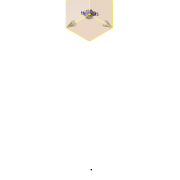
# Autodesk Inventor part: CounterWeightFixation_oldVersion
Saved by Autodesk Inventor 2021.4 (Build 254397000, 397)
## iProperties
Created: 2022-07-01
Part Number: CounterWeightFixation_oldVersion
Material: PAEK Plastic
Document SubType Name: Modeling
Designer: alexw
Density: 0.206549 g/cm^3
Appearance: Smooth - White
Mass: 22 g
Surface Area: 255.397 cm^2
Volume: 106.513 cm^3
Author: alexw
Autodesk Inventor part; units mm, degrees
ref_plane "YZ Plane" through (0, 0, 0) normal (1, 0, 0) x (0, 1, 0)
ref_plane "XZ Plane" through (0, 0, 0) normal (0, 1, 0) x (-1, 0, 0)
ref_plane "XY Plane" through (0, 0, 0) normal (0, 0, 1) x (1, 0, 0)
sketch "Sketch1" plane through (0, 0, 0) normal (0, 0, 1) x (1, 0, 0)
  arc A0 (0, 30) -> (0, -30) centre (0, 0) ccw
  arc A1 (0, 17.5) -> (0, -17.5) centre (0, 0) ccw
  line L0 (0, 36.2) -> (0, -36.2) construction
  line L1 (0, 17.5) -> (0, 36.2) construction
  line L2 (0, -17.5) -> (0, -36.2) construction
  circle A2 centre (-74.9655, 11.8734) radius 20.1
  circle A3 centre (0, 0) radius 75.9 construction
  arc A4 (0, 23.75) -> (0, -23.75) centre (0, 0) ccw construction
  line L3 (0, -23.75) -> (0, 23.75) construction
  line L4 (0, 23.75) -> (0, 0) construction
  arc A5 (0, 17.5) -> (0, 36.2) centre (0, 26.85) ccw
  arc A6 (0, -36.2) -> (0, -17.5) centre (0, -26.85) ccw
  arc A7 (-75.423, 35.4689) -> (-88.8905, -7.1807) centre (-74.9655, 11.8734) ccw
  line L5 (0, 30) -> (8.8034, 30)
  line L6 (0, -30) -> (8.8034, -30)
  arc A8 (0, 36.2) -> (0, -36.2) centre (0, 0) ccw
  circle A9 centre (-74.9655, 11.8734) radius 23.6 construction
  arc A10 (0, 36.2) -> (-75.423, 35.4689) centre (0, -3854.8474) ccw
  arc A11 (-88.8905, -7.1807) -> (0, -36.2) centre (0, 114.4519) ccw
  line L7 (0, 0) -> (-75.9, 0) construction
  line L8 (-74.9655, 11.8734) -> (0, 0) construction
  line L9 (0, 0) -> (-75.0466, 11.3497) construction
  point P0 (-23.75, 0)
  dimension "d0" = 60
  dimension "d1" = 35
  dimension "d2" = 75.9
  dimension "d5" = 40.2
  dimension "FixHole_Rad" = 23.75
  dimension "d25" = 72.4
  dimension "d52" = 3.5
  dimension "d63" = 0
  dimension "d72" = 9
  dimension "d73" = 8.6
  constraints: 27 point on circle, 20 end point, 12 centre point, 8 point on line, 7 coincident, 5 tangent, 4 midpoint, 3 vertical, 1 collinear, 1 concentric, 1 horizontal, 1 perpendicular, 2 other
  measures "d0" diameter of A0
  measures "d1" diameter of A1
  measures "d2" radius of A3
  measures "d5" diameter of A2
  measures "FixHole_Rad" radius of A4
  measures "d25" diameter of A8
  measures "d52" radial gap between concentric circles of A9 A2
  measures "d63" distance of A9.centre L8.start
  measures "d72" angle of L8 L7
  measures "d73" angle of L9 L7
extrude "Extrusion1" add sketch "Sketch1" along normal blind 30 contours L5 A5 A1 A6 L6 A0 | A0 L6 A6 A8 A5 L5 | A8 A11 A7 A10 | A2
extrude "Extrusion3" cut sketch "Sketch1" along normal blind 20 contours L5 A5 A1 A6 L6 A0
extrude "Extrusion5" cut sketch "Sketch1" along normal blind 26.6 contours A2
extrude "Extrusion6" cut sketch "Sketch1" against normal blind 0.4 from surface at 30 contours A2
extrude "Extrusion8" cut sketch "Sketch1" against normal blind 2 from surface at 30 contours L5 A5 A1 A6 L6 A0 | A0 L6 A6 A8 A5 L5
sketch "Sketch2" plane through (0, 0, 28) normal (0, 0, 1) x (1, 0, 0)
  point P0 (0, 0)
  point P1 (0, -23.75)
  point P2 (-23.75, 0)
  point P3 (0, 23.75)
hole "Hole2" at (0, -23.75, 28) at (-23.75, 0, 28) at (0, 23.75, 28) direction (0, 0, -1) diameter 4.5 end through all counterbore diameter 8 counterbore depth 4.6 clearance for "Socket Head Cap Screw ISO 4762" size "M4" standard "ISO"
fillet "Fillet1" radius 8 3 edges at (-88.8905, -7.1807, 15) (0, 36.2, 29) (0, -36.2, 29)
hole "Hole3" at (0, -23.75, 0) at (-23.75, 0, 0) direction (0, 0, 1) diameter 5.3 end through all clearance for "Countersunk Flat Head Screw DIN EN ISO 2009" size "M5" standard "DIN"
hole "Hole4" at (-74.9655, 11.8734, 0) direction (0, 0, 1) diameter 4.3 end through all clearance for "Countersunk Flat Head Screw DIN EN ISO 2009" size "M4" standard "DIN"
equation "\"d0\" = SJ_D_out"
equation "\"d12\" = d11"
equation "\"d13\" = d12"
equation "\"StabelizerExtrusion\" = 8"
equation "\"SJ_D_out\" = 60"
equation "\"d11\" = 3.8"
body "Solid1"
